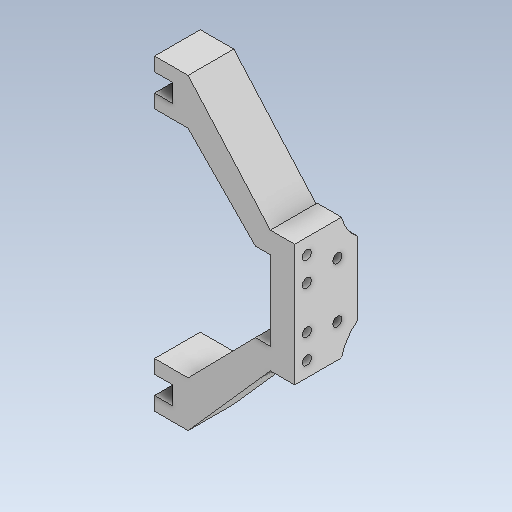
# Autodesk Inventor part: body_carbon_fiber_holder_1
Saved by Autodesk Inventor 2020 (Build 240168000, 168)
## iProperties
Created: 2019-07-16
Part Number: body_carbon_fiber_holder_1
Material: Generic
Document SubType Name: Modeling
Designer: psrob
Density: 1 g/cm^3
Appearance: Default
Author: psrob
Autodesk Inventor part; units mm, degrees
ref_plane "YZ Plane" through (0, 0, 0) normal (1, 0, 0) x (0, 1, 0)
ref_plane "XZ Plane" through (0, 0, 0) normal (0, 1, 0) x (-1, 0, 0)
ref_plane "XY Plane" through (0, 0, 0) normal (0, 0, 1) x (1, 0, 0)
sketch "Sketch1" plane through (0, 0, 0) normal (0, 0, 1) x (1, 0, 0)
  line L0 (-56, -67.5) -> (-50, -67.5) projected
  line L1 (-56, -73.5) -> (-56, -67.5) projected
  line L2 (-50, -73.5) -> (-56, -73.5) projected
  line L3 (-50, -67.5) -> (-50, -73.5) projected
  circle A0 centre (-53, -70.5) radius 2 projected
  line L4 (-56, 18.5) -> (-50, 18.5) projected
  line L5 (-56, 12.5) -> (-56, 18.5) projected
  line L6 (-50, 12.5) -> (-56, 12.5) projected
  line L7 (-50, 18.5) -> (-50, 12.5) projected
  circle A1 centre (-53, 15.5) radius 2 projected
  line L8 (-10, -47.5) -> (-10, -7.5) projected
  line L9 (-10, -47.5) -> (-18, -47.5)
  line L10 (-18, -47.5) -> (-18, -7.5)
  line L11 (-18, -7.5) -> (-10, -7.5)
  line L12 (-10, -7.5) -> (-10, -47.5)
  line L13 (-56, -78) -> (-56, -63)
  line L14 (-56, -63) -> (-50, -63)
  line L15 (-50, -63) -> (-50, -78)
  line L16 (-50, -78) -> (-56, -78)
  line L17 (-56, -78) -> (-50, -63) construction
  line L18 (-56, -63) -> (-50, -78) construction
  line L19 (-56, 8) -> (-56, 23)
  line L20 (-56, 23) -> (-50, 23)
  line L21 (-50, 23) -> (-50, 8)
  line L22 (-50, 8) -> (-56, 8)
  line L23 (-56, 8) -> (-50, 23) construction
  line L24 (-56, 23) -> (-50, 8) construction
  line L25 (-18, -47.5) -> (-18, -35.5)
  line L26 (-18, -7.5) -> (-18, -19.5)
  line L27 (-50, -78) -> (-45, -78)
  line L28 (-45, -78) -> (-45, -63)
  line L29 (-45, -63) -> (-50, -63)
  line L30 (-50, -63) -> (-50, -78)
  line L31 (-50, 23) -> (-45, 23)
  line L32 (-45, 23) -> (-45, 8)
  line L33 (-45, 8) -> (-50, 8)
  line L34 (-50, 8) -> (-50, 23)
  line L35 (-45, -63) -> (-18, -35.5)
  line L36 (-45, -78) -> (-18, -47.5)
  line L37 (-18, -19.5) -> (-45, 8)
  line L38 (-18, -7.5) -> (-45, 23)
  point P0 (0, 0)
  dimension "d0" = 8
  dimension "d1" = 40
  dimension "d2" = 15
  dimension "d3" = 6
  dimension "d4" = 15
  dimension "d5" = 6
  dimension "d6" = 12
  dimension "d7" = 12
  dimension "d8" = 5
  dimension "d9" = 15
  dimension "d10" = 5
  dimension "d11" = 15
  constraints: 60 end point, 10 parallel, 5 perpendicular, 4 midpoint, 3 horizontal, 2 point on line, 2 vertical
  measures "d0" distance of L10.end L11.end
  measures "d1" distance of L9.end L10.end
  measures "d2" distance of L13.start L13.end
  measures "d3" distance of L13.end L14.end
  measures "d4" distance of L19.start L19.end
  measures "d5" distance of L19.end L20.end
  measures "d6" distance of L9.end L25.end
  measures "d7" distance of L10.end L26.end
  measures "d8" distance of L29.end L28.end
  measures "d9" distance of L28.end L27.end
  measures "d10" distance of L32.end L33.end
  measures "d11" distance of L31.end L32.end
extrude "Extrusion1" add sketch "Sketch1" against normal blind 15 contours L13 L14 L15 L0 | L15 L29 L28 L27 L3 | L2 L15 L16 L13 | L35 L10 L36 L28 | L10 L11 L8 L9 | L37 L32 L38 L10 | L33 L21 L7 L31 L32 | L22 L19 L6 L21 | L21 L4 L19 L20
sketch "Sketch2" plane through (-18, -35.5, 0) normal (-1, 0, 0) x (0, 0, 1)
  circle A0 centre (-59, 1) radius 1.5 projected
  circle A1 centre (-59, 15) radius 1.5 projected
  circle A2 centre (-69, 15) radius 1.5 projected
  circle A3 centre (-69, 1) radius 1.5 projected
  circle A4 centre (-19, 8) radius 1.5 projected
  circle A5 centre (-69, 8) radius 1.5 projected
  circle A6 centre (-79, 8) radius 1.5 projected
  circle A7 centre (-59, 8) radius 1.5 projected
  circle A8 centre (-9, 8) radius 1.5 projected
  line L0 (-86.8834, 23) -> (-82.7232, 25.2265) projected
  line L1 (-86.8834, 23) -> (-86.8834, -7) projected
  line L2 (-82.7232, -9.2265) -> (-86.8834, -7) projected
  line L3 (-82.7232, -9.2265) -> (-71.8834, -2) projected
  line L4 (-71.8834, -2) -> (-54.8834, -2) projected
  line L5 (-54.8834, -2) -> (-54.8834, 2) projected
  arc A9 (-51.8834, 5) -> (-54.8834, 2) centre (-51.8834, 2) ccw projected
  line L6 (-51.8834, 5) -> (-28.9711, 5) projected
  arc A10 (-25.9711, 2) -> (-28.9711, 5) centre (-28.9711, 2) ccw projected
  line L7 (-25.9711, 2) -> (-25.9711, -0.0217) projected
  line L8 (-25.9711, -0.0217) -> (-20.6, -4.05) projected
  arc A11 (-15.3825, -12) -> (-20.6, -4.05) centre (-29, -15.25) ccw projected
  line L9 (-15.3825, -12) -> (0, -12) projected
  line L10 (0, -12) -> (0, 28) projected
  line L11 (0, 28) -> (-15.3825, 28) projected
  arc A12 (-20.6, 20.05) -> (-15.3825, 28) centre (-29, 31.25) ccw projected
  line L12 (-20.6, 20.05) -> (-25.9711, 16.0217) projected
  line L13 (-25.9711, 16.0217) -> (-25.9711, 14) projected
  arc A13 (-28.9711, 11) -> (-25.9711, 14) centre (-28.9711, 14) ccw projected
  line L14 (-28.9711, 11) -> (-51.8834, 11) projected
  arc A14 (-54.8834, 14) -> (-51.8834, 11) centre (-51.8834, 14) ccw projected
  line L15 (-54.8834, 14) -> (-54.8834, 18) projected
  line L16 (-54.8834, 18) -> (-71.8834, 18) projected
  line L17 (-71.8834, 18) -> (-82.7232, 25.2265) projected
  circle A15 centre (-81.8834, -2) radius 1.5 projected
  circle A16 centre (-4, 1) radius 1.5 projected
  circle A17 centre (-14, -1) radius 1.5 projected
  circle A18 centre (-4, -7) radius 1.5 projected
  circle A19 centre (-14, 17) radius 1.5 projected
  circle A20 centre (-4, 15) radius 1.5 projected
  circle A21 centre (-4, 23) radius 1.5 projected
  circle A22 centre (-81.8834, 18) radius 1.5 projected
  line L18 (-20.6, 20.05) -> (-20.6, -4.05)
  point P0 (0, 35.5)
  constraints: 2 end point, 1 vertical
extrude "Extrusion2" add sketch "Sketch2" against normal up to surface (8 mm away) contours A4 | A12 L11 L10 L9 A11 L18 | A17 | A19
sketch "Sketch3" plane through (-18, -35.5, 0) normal (-1, 0, 0) x (0, 0, 1)
  circle A0 centre (-4, 1) radius 1.5 projected
  circle A1 centre (-4, -7) radius 1.5 projected
  circle A2 centre (-14, -1) radius 1.5 projected
  circle A3 centre (-14, 17) radius 1.5 projected
  circle A4 centre (-4, 23) radius 1.5 projected
  circle A5 centre (-4, 15) radius 1.5 projected
  point P0 (0, 35.5)
extrude "Extrusion3" cut sketch "Sketch3" along normal mid plane 30
sketch "Sketch4" plane through (0, 0, -15) normal (0, 0, -1) x (-1, 0, 0)
  line L0 (18, -17.382) -> (20.0795, -17.382) projected
  line L1 (20.0795, -17.382) -> (45, 8) projected
  line L2 (45, 8) -> (56, 8) projected
  line L3 (56, 8) -> (56, 12.5) projected
  line L4 (56, 12.5) -> (50, 12.5) projected
  line L5 (50, 12.5) -> (50, 18.5) projected
  line L6 (50, 18.5) -> (56, 18.5) projected
  line L7 (56, 18.5) -> (56, 23) projected
  line L8 (56, 23) -> (45, 23) projected
  line L9 (45, 23) -> (18, -7.5) projected
  line L10 (18, -7.5) -> (18, -17.382) projected
  line L11 (20.0795, -37.618) -> (18, -37.618) projected
  line L12 (18, -37.618) -> (18, -47.5) projected
  line L13 (18, -47.5) -> (45, -78) projected
  line L14 (45, -78) -> (56, -78) projected
  line L15 (56, -78) -> (56, -73.5) projected
  line L16 (56, -73.5) -> (50, -73.5) projected
  line L17 (50, -73.5) -> (50, -67.5) projected
  line L18 (50, -67.5) -> (56, -67.5) projected
  line L19 (56, -67.5) -> (56, -63) projected
  line L20 (56, -63) -> (45, -63) projected
  line L21 (45, -63) -> (20.0795, -37.618) projected
  line L22 (18, -7.5) -> (18, -17.382) projected
  line L23 (18, -7.5) -> (18, -14.5)
  line L24 (18, -37.618) -> (18, -47.5) projected
  line L25 (18, -47.5) -> (18, -40.5)
  line L26 (18, -14.5) -> (30, -14.5)
  line L27 (30, -14.5) -> (30, -40.5)
  line L28 (30, -40.5) -> (18, -40.5)
  line L29 (18, -40.5) -> (18, -14.5)
  point P0 (0, 0)
  dimension "d18" = 7
  dimension "d19" = 7
  dimension "d20" = 12
  dimension "d21" = 26
  constraints: 12 end point, 2 parallel, 2 point on line, 1 horizontal, 1 perpendicular
  measures "d18" distance of L9.end L23.end
  measures "d19" distance of L12.end L25.end
  measures "d20" distance of L27.end L28.end
  measures "d21" distance of L26.end L27.end
extrude "Extrusion4" cut sketch "Sketch4" against normal blind 30 contours L10 L26 L1 L0 | L0 L1 L26 L27 L28 L21 L11 L29 | L11 L21 L28 L12
body "Solid1"
